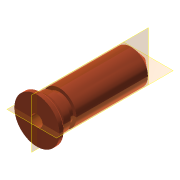
# Autodesk Inventor part: nozzle0.8
Saved by Autodesk Inventor 2016 (Build 200138000, 138)
## iProperties
Created: 2016-01-20
Part Number: nozzle0.8
Material: Copper
Document SubType Name: Modeling
Designer: admin
Density: 1 g/cm^3
Appearance: Copper - Satin
Author: admin
Autodesk Inventor part; units mm, degrees
ref_plane "XZ Plane" through (0, 0, 0) normal (0, 1, 0) x (-1, 0, 0)
sketch "Sketch1" plane through (0, 0, 0) normal (0, 1, 0) x (-1, 0, 0)
  circle A0 centre (0, 0) radius 4
  dimension "d0" = 8
  constraints: 1 centre point, 1 coincident
  measures "d0" diameter of A0
extrude "Extrusion1" add sketch "Sketch1" along normal blind 1
sketch "Sketch2" plane through (0, 1, 0) normal (0, 1, 0) x (1, 0, 0)
  circle A0 centre (0, 0) radius 4 projected
  circle A1 centre (0, 0) radius 3
  dimension "d3" = 6
  constraints: 1 centre point, 1 coincident
  measures "d3" diameter of A1
extrude "Extrusion2" add sketch "Sketch2" along normal blind 15.668 contours A1
sketch "Sketch3" plane through (0, 0, 0) normal (0, -1, 0) x (1, 0, 0)
  circle A0 centre (0, 0) radius 4 projected
  circle A1 centre (0, 0) radius 1
  dimension "d6" = 2
  constraints: 1 centre point, 1 coincident
  measures "d6" diameter of A1
extrude "Extrusion3" cut sketch "Sketch3" against normal blind 21 contours A1
sketch "Sketch4" plane through (0, 0, 0) normal (1, 0, 0) x (0, 1, 0)
  line L0 (1, 3) -> (16.668, 3) projected
  line L1 (1, -3) -> (16.668, -3) projected
  line L2 (0, 0) -> (17, 0)
  line L3 (16.668, 3) -> (18.9755, 0.25)
  line L4 (16.668, -3) -> (16.668, 3) projected
  line L5 (16.668, 0.2) -> (18.9755, 0.2)
  line L6 (17.7072, 0.4) -> (16.668, 1)
  line L7 (0, 1) -> (16.668, 1) projected
  line L8 (16.668, 1) -> (16.668, 3)
  line L9 (18.9755, 0.25) -> (18.9755, 0.2)
  line L10 (17.7072, 0.4) -> (18.8077, 0.4)
  line L11 (18.8077, 0.4) -> (18.8077, 0.45)
  point P0 (17.8856, 0.2)
  dimension "d9" = 40
  dimension "d10" = 0.2
  dimension "d11" = 30
  dimension "d20" = 0.05
  dimension "d21" = 0.4
  dimension "d22" = 0.05
  constraints: 16 end point, 5 point on line, 3 perpendicular, 1 parallel
  measures "d9" angle of L4 L3
  measures "d10" distance between parallel lines of L2 L5
  measures "d11" angle of L5 L6
  measures "d20" distance of L5.end L3.end
  measures "d21" distance between parallel lines of L2 L10
  measures "d22" distance of L10.end L11.end
revolve "Revolution1" add sketch "Sketch4" angle 360 about axis through (0, 0, 0) along (0, 1, 0) contours L3 L11 L10 L6 L4
sketch "Sketch5" plane through (0, 0, 0) normal (0, 0, 1) x (1, 0, 0)
  circle A0 centre (3, 1.35) radius 0.35
  line L0 (4, 1) -> (-4, 1) projected
  line L1 (3, 3) -> (3, 0)
  line L2 (0, 1.1204) -> (0, 3)
  line L3 (2.7525, 1.5975) -> (3.3734, 2.2184)
  line L4 (3.3734, 2.2184) -> (3.3499, 1.3406)
  point P0 (0, 0)
  dimension "d14" = 0.7
  dimension "d19" = 45
  constraints: 8 end point, 3 tangent, 2 point on circle, 1 centre point, 1 point on line, 1 vertical, 2 other
  measures "d14" diameter of A0
  measures "d19" angle of L0 L3
revolve "Revolution2" cut sketch "Sketch5" angle 360 about axis through (0, 1.1204, 0) along (0, 1, 0)
chamfer "Chamfer1" distance 0.3 angle 45 1 edges at (4, 1, 0)
sketch "Sketch6" plane through (0, 0, 0) normal (0, 0, 1) x (1, 0, 0)
  line L0 (-3, 1.845) -> (-3, 16.668) projected
  line L1 (-3, 3) -> (-2.4, 3)
  line L2 (-2.4, 3) -> (-2.4, 4)
  line L3 (-2.4, 4) -> (-3, 4)
  line L4 (-3, 4) -> (-3, 3)
  line L5 (-4, 0) -> (4, 0) projected
  line L6 (0, 0) -> (0, -2.0894)
  dimension "d23" = 0.6
  dimension "d24" = 1
  dimension "d25" = 3
  constraints: 10 end point, 2 parallel, 1 horizontal, 1 perpendicular, 1 point on line, 1 vertical
  measures "d23" distance of L3.end L2.end
  measures "d24" distance of L2.end L1.end
  measures "d25" distance between parallel lines of L5 L1
revolve "Revolution3" cut sketch "Sketch6" angle 360 about axis through (0, 0, 0) along (0, -1, 0)
body "Solid1"
